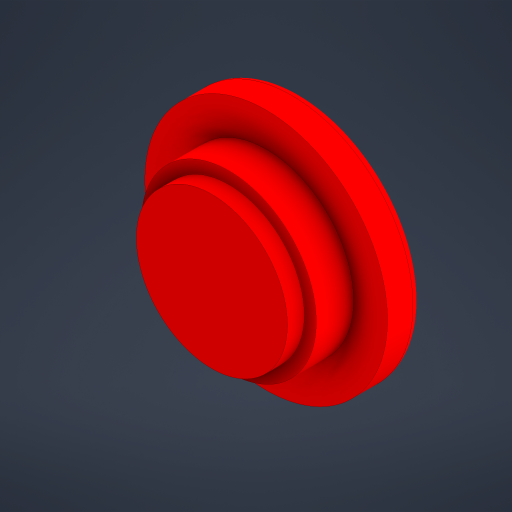
# Autodesk Inventor part: Inner Ring Press
Saved by Autodesk Inventor 2023.4 (Build 274418000, 418)
## iProperties
Created: 2024-07-23
Part Number: Inner Ring Press
Material: Generic
Document SubType Name: Modeling
Designer: xSibe
Density: 1 g/cm^3
Appearance: Plastic Red
Author: xSibe
Autodesk Inventor part; units mm, degrees
ref_plane "YZ Plane" through (0, 0, 0) normal (1, 0, 0) x (0, 1, 0)
ref_plane "XZ Plane" through (0, 0, 0) normal (0, 1, 0) x (-1, 0, 0)
ref_plane "XY Plane" through (0, 0, 0) normal (0, 0, 1) x (1, 0, 0)
sketch "Sketch1" plane through (0, 0, 0) normal (0, 0, 1) x (1, 0, 0)
  circle A0 centre (0, 0) radius 11.125
  circle A1 centre (0, 0) radius 12.875
  circle A2 centre (0, 0) radius 17.875
  dimension "d0" = 22.25
  dimension "d1" = 25.75
  dimension "d2" = 5
  constraints: 3 centre point, 2 coincident
  measures "d0" diameter of A0
  measures "d1" diameter of A1
  measures "d2" radial gap between concentric circles of A1 A2
extrude "Extrusion1" add sketch "Sketch1" along normal blind 5 contours A0 | A1 | A2
extrude "Extrusion2" add sketch "Sketch1" along normal blind 5.5 from surface at 5 contours A0 | A1
extrude "Extrusion3" add sketch "Sketch1" along normal blind 2.5 from surface at 10.5 contours A0
fillet "Fillet1" radius 1.25 1 edges at (-17.875, 0, 0)
sketch "Sketch2" plane through (0, 0, 0) normal (0, 0, -1) x (-1, 0, 0)
  line L0 (-12.5, -12.5) -> (12.5, -12.5)
  line L1 (12.5, -12.5) -> (12.5, 12.5)
  line L2 (12.5, 12.5) -> (-12.5, 12.5)
  line L3 (-12.5, 12.5) -> (-12.5, -12.5)
  line L4 (-12.5, -12.5) -> (12.5, 12.5) construction
  line L5 (12.5, -12.5) -> (-12.5, 12.5) construction
  line L6 (-12.5, 12.5) -> (12.5, 12.5) construction
  line L7 (12.5, 12.5) -> (12.5, -12.5) construction
  line L8 (12.5, -12.5) -> (-12.5, -12.5) construction
  line L9 (-12.5, -12.5) -> (-12.5, 12.5) construction
  line L10 (3.8655, -10) -> (-3.8817, -10)
  line L11 (-3.8817, -10) -> (-3.8817, -7.9579)
  line L12 (-3.8817, -7.9579) -> (-1.3371, -7.9579)
  line L13 (-1.3371, -7.9579) -> (-1.3371, 7.9579)
  line L14 (-1.3371, 7.9579) -> (-3.8817, 7.9579)
  line L15 (-3.8817, 7.9579) -> (-3.8817, 10)
  line L16 (-3.8817, 10) -> (3.8655, 10)
  line L17 (3.8655, 10) -> (3.8655, 7.9579)
  line L18 (3.8655, 7.9579) -> (1.3209, 7.9579)
  line L19 (1.3209, 7.9579) -> (1.3209, -7.9579)
  line L20 (1.3209, -7.9579) -> (3.8655, -7.9579)
  line L21 (3.8655, -7.9579) -> (3.8655, -10)
  point P0 (0, 0)
  dimension "d10" = 25
  dimension "d11" = 25
  constraints: 12 end point, 2 coincident, 2 midpoint, 2 parallel, 1 horizontal, 1 perpendicular, 2 other
  measures "d10" distance of L2.end L1.end
  measures "d11" distance of L1.end L0.end
extrude "Extrusion4" cut sketch "Sketch2" against normal blind 0.25 contours L10 L11 L12 L13 L14 L15 L16 L17 L18 L19 L20 L21
chamfer "Chamfer1" distance 0.25 angle 45 12 edges at (0.0081, -10, 0.25) (3.8817, -8.9789, 0.25) (2.6094, -7.9579, 0.25) (1.3371, 0, 0.25) (2.6094, 7.9579, 0.25) (3.8817, 8.9789, 0.25) (0.0081, 10, 0.25) (-3.8655, 8.9789, 0.25) (-2.5932, 7.9579, 0.25) (-1.3209, 0, 0.25) (-2.5932, -7.9579, 0.25) (-3.8655, -8.9789, 0.25)
body "Solid1"
